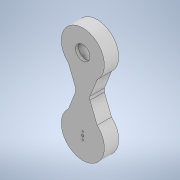
# Autodesk Inventor part: 2ndArm
Saved by Autodesk Inventor 2022 (Build 260153000, 153)
## iProperties
Created: 2022-02-11
Part Number: 2ndArm
Material: Generic
Document SubType Name: Modeling
Designer: Alexa
Density: 1 g/cm^3
Appearance: Default
Author: Alexa
Autodesk Inventor part; units mm, degrees
ref_plane "YZ Plane" through (0, 0, 0) normal (1, 0, 0) x (0, 1, 0)
ref_plane "XZ Plane" through (0, 0, 0) normal (0, 1, 0) x (-1, 0, 0)
ref_plane "XY Plane" through (0, 0, 0) normal (0, 0, 1) x (1, 0, 0)
sketch "Sketch1" plane through (0, 0, 0) normal (0, 0, 1) x (1, 0, 0)
  circle A0 centre (0, 0) radius 30
  circle A1 centre (0, 100) radius 30
  line L0 (-20, 0) -> (20, 0)
  line L1 (20, 0) -> (20, 100)
  line L2 (20, 100) -> (-20, 100)
  line L3 (-20, 100) -> (-20, 0)
  point P0 (20, 77.6393)
  point P1 (-20, 77.6393)
  point P2 (-20, 22.3607)
  point P3 (20, 22.3607)
  dimension "d0" = 60
  dimension "d1" = 60
  dimension "d2" = 40
  constraints: 8 end point, 2 centre point, 2 parallel, 1 coincident, 1 horizontal, 1 perpendicular
  measures "d0" diameter of A0
  measures "d1" diameter of A1
  measures "d2" distance of L2.end L1.end
extrude "Extrusion1" add sketch "Sketch1" along normal blind 20
sketch "Sketch2" plane through (0, 0, 20) normal (0, 0, 1) x (1, 0, 0)
  circle A0 centre (0, 0) radius 10
  dimension "d5" = 20
  constraints: 1 centre point, 1 coincident
  measures "d5" diameter of A0
extrude "Extrusion2" cut sketch "Sketch2" against normal blind 16
sketch "Sketch3" plane through (0, 0, 4) normal (0, 0, 1) x (1, 0, 0)
  circle A0 centre (0, 0) radius 1
  circle A1 centre (5, 0) radius 1
  circle A2 centre (-5, 0) radius 1
  dimension "d11" = 2
  dimension "d12" = 2
  dimension "d13" = 2
  constraints: 3 centre point, 1 coincident
  measures "d11" diameter of A0
  measures "d12" diameter of A1
  measures "d13" diameter of A2
extrude "Extrusion3" cut sketch "Sketch3" against normal blind 28.45
sketch "Sketch4" plane through (0, 0, 0) normal (0, 0, -1) x (-1, 0, 0)
  line L0 (0, 100) -> (10, 100)
  line L1 (10, 100) -> (10, 70)
  line L2 (10, 70) -> (0, 70)
  line L3 (0, 70) -> (0, 100)
  line L4 (0, 100) -> (-10, 100)
  line L5 (-10, 100) -> (-10, 70)
  line L6 (-10, 70) -> (0, 70)
  line L7 (0, 70) -> (0, 100)
  line L8 (10, 100) -> (-10, 100)
  line L9 (-10, 100) -> (-10, 110.5)
  line L10 (-10, 110.5) -> (10, 110.5)
  line L11 (10, 110.5) -> (10, 100)
  point P0 (0, 0)
  dimension "d16" = 10
  dimension "d17" = 30
  dimension "d18" = 10
  dimension "d19" = 10.5
  constraints: 24 end point, 6 parallel, 3 horizontal, 3 perpendicular, 2 point on line
  measures "d16" distance of L1.end L2.end
  measures "d17" distance of L0.end L1.end
  measures "d18" distance of L6.end L5.end
  measures "d19" distance of L8.end L9.end
extrude "Extrusion4" cut sketch "Sketch4" against normal blind 16
sketch "Sketch5" plane through (0, 0, 0) normal (0, 0, -1) x (-1, 0, 0)
  line L0 (10, 110.5) -> (10, 70) projected
  line L1 (10, 110.5) -> (-10, 110.5)
  line L2 (-10, 110.5) -> (-10, 118.1)
  line L3 (-10, 118.1) -> (10, 118.1)
  line L4 (10, 118.1) -> (10, 110.5)
  line L5 (10, 70) -> (-10, 70)
  line L6 (-10, 70) -> (-10, 62.4)
  line L7 (-10, 62.4) -> (10, 62.4)
  line L8 (10, 62.4) -> (10, 70)
  line L9 (-10, 110.5) -> (10, 110.5) projected
  line L10 (10, 110.5) -> (-10, 110.5)
  line L11 (-10, 110.5) -> (-10, 114.6)
  line L12 (-10, 114.6) -> (10, 114.6)
  line L13 (10, 114.6) -> (10, 110.5)
  line L14 (10, 70) -> (-10, 70)
  line L15 (-10, 70) -> (-10, 65.9)
  line L16 (-10, 65.9) -> (10, 65.9)
  line L17 (10, 65.9) -> (10, 70)
  line L18 (0, 110.5) -> (5, 110.5)
  line L19 (5, 110.5) -> (5, 114.6)
  line L20 (5, 114.6) -> (0, 114.6)
  line L21 (0, 114.6) -> (0, 110.5)
  line L22 (0, 110.5) -> (-5, 110.5)
  line L23 (-5, 110.5) -> (-5, 114.6)
  line L24 (-5, 114.6) -> (0, 114.6)
  line L25 (0, 114.6) -> (0, 110.5)
  line L26 (0, 70) -> (5, 70)
  line L27 (5, 70) -> (5, 65.9)
  line L28 (5, 65.9) -> (0, 65.9)
  line L29 (0, 65.9) -> (0, 70)
  line L30 (0, 70) -> (-5, 70)
  line L31 (-5, 70) -> (-5, 65.9)
  line L32 (-5, 65.9) -> (0, 65.9)
  line L33 (0, 65.9) -> (0, 70)
  point P0 (0, 0)
  dimension "d22" = 7.6
  dimension "d23" = 7.6
  dimension "d24" = 4.1
  dimension "d25" = 4.1
  dimension "d26" = 5
  dimension "d27" = 5
  dimension "d28" = 5
  dimension "d29" = 5
  constraints: 64 end point, 16 parallel, 8 horizontal, 8 perpendicular, 7 point on line, 2 midpoint
  measures "d22" distance of L1.end L2.end
  measures "d23" distance of L6.end L5.end
  measures "d24" distance of L10.end L11.end
  measures "d25" distance of L15.end L14.end
  measures "d26" distance of L20.end L19.end
  measures "d27" distance of L23.end L24.end
  measures "d28" distance of L27.end L28.end
  measures "d29" distance of L32.end L31.end
extrude "Extrusion5" cut sketch "Sketch5" against normal blind 10
sketch "Sketch6" plane through (0, 0, 10) normal (0, 0, -1) x (-1, 0, 0)
  line L0 (10, 110.5) -> (10, 70) projected
  line L1 (-10, 62.4) -> (-10, 118.1) projected
  line L2 (10, 110.5) -> (-10, 110.5)
  line L3 (-10, 110.5) -> (-10, 114.6)
  line L4 (-10, 114.6) -> (10, 114.6)
  line L5 (10, 114.6) -> (10, 110.5)
  line L6 (10, 70) -> (-10, 70) projected
  line L7 (-10, 62.4) -> (-10, 70) projected
  line L8 (10, 70) -> (-10, 70)
  line L9 (-10, 70) -> (-10, 65.9)
  line L10 (-10, 65.9) -> (10, 65.9)
  line L11 (10, 65.9) -> (10, 70)
  line L12 (-10, 110.5) -> (10, 110.5) projected
  line L13 (0, 114.6) -> (5, 114.6)
  line L14 (5, 114.6) -> (5, 110.5)
  line L15 (5, 110.5) -> (0, 110.5)
  line L16 (0, 110.5) -> (0, 114.6)
  line L17 (0, 110.5) -> (-5, 110.5)
  line L18 (-5, 110.5) -> (-5, 114.6)
  line L19 (-5, 114.6) -> (0, 114.6)
  line L20 (0, 114.6) -> (0, 110.5)
  line L21 (0, 70) -> (5, 70)
  line L22 (5, 70) -> (5, 65.9)
  line L23 (5, 65.9) -> (0, 65.9)
  line L24 (0, 65.9) -> (0, 70)
  line L25 (0, 70) -> (-5, 70)
  line L26 (-5, 70) -> (-5, 65.9)
  line L27 (-5, 65.9) -> (0, 65.9)
  line L28 (0, 65.9) -> (0, 70)
  circle A0 centre (5, 114.6) radius 1.35
  circle A1 centre (-5, 114.6) radius 1.35
  circle A2 centre (5, 65.9) radius 1.35
  circle A3 centre (-5, 65.9) radius 1.35
  point P0 (0, 0)
  dimension "d32" = 4.1
  dimension "d33" = 4.1
  dimension "d34" = 5
  dimension "d35" = 5
  dimension "d36" = 2.7
  dimension "d37" = 2.7
  dimension "d38" = 2.7
  dimension "d39" = 2.7
  constraints: 48 end point, 12 parallel, 8 point on line, 6 horizontal, 6 perpendicular, 4 centre point, 4 coincident, 2 midpoint
  measures "d32" distance of L2.end L3.end
  measures "d33" distance of L9.end L8.end
  measures "d34" distance of L14.end L15.end
  measures "d35" distance of L18.end L19.end
  measures "d36" diameter of A0
  measures "d37" diameter of A1
  measures "d38" diameter of A2
  measures "d39" diameter of A3
extrude "Extrusion6" cut sketch "Sketch6" against normal blind 8 contours A0 L4 L14 | L14 L4 A0 | L4 A0 | A2 L10 L22 | L22 L10 A2 | A2 L10 | A1 L4 L18 | L18 L4 A1 | L4 A1 | A3 L10 L26 | L26 L10 A3 | A3 L10
sketch "Sketch7" plane through (0, 0, 20) normal (0, 0, 1) x (1, 0, 0)
  circle A0 centre (0, 100) radius 10
  point P0 (0, 0)
  dimension "d50" = 20
  constraints: 1 centre point
  measures "d50" diameter of A0
extrude "Extrusion7" cut sketch "Sketch7" against normal blind 4
sketch "Sketch8" plane through (0, 0, 0) normal (0, 0, -1) x (-1, 0, 0)
  line L0 (20, 77.6393) -> (20, 22.3607) projected
  arc A0 (20, 77.6393) -> (-20, 77.6393) centre (0, 100) ccw projected
  line L1 (20, 22.3607) -> (-20, 22.3607)
  line L2 (-20, 22.3607) -> (-20, 77.6393)
  line L3 (-20, 77.6393) -> (20, 77.6393)
  line L4 (20, 77.6393) -> (20, 22.3607)
  line L5 (10, 118.1) -> (10, 62.4) projected
  line L6 (10, 77.6393) -> (-10, 77.6393)
  line L7 (-10, 77.6393) -> (-10, 47.6393)
  line L8 (-10, 47.6393) -> (10, 47.6393)
  line L9 (10, 47.6393) -> (10, 77.6393)
  line L10 (-10, 22.3607) -> (10, 22.3607)
  line L11 (10, 22.3607) -> (10, 52.3607)
  line L12 (10, 52.3607) -> (-10, 52.3607)
  line L13 (-10, 52.3607) -> (-10, 22.3607)
  line L14 (20, 77.6393) -> (10, 52.3607)
  line L15 (10, 47.6393) -> (20, 22.3607)
  line L16 (-20, 77.6393) -> (-10, 52.3607)
  line L17 (-10, 47.6393) -> (-20, 22.3607)
  point P0 (0, 0)
  dimension "d53" = 20
  dimension "d54" = 30
  dimension "d55" = 30
  constraints: 32 end point, 6 parallel, 5 point on line, 3 horizontal, 3 perpendicular
  measures "d53" distance of L8.end L7.end
  measures "d54" distance of L7.end L6.end
  measures "d55" distance of L11.end L10.end
extrude "Extrusion8" cut sketch "Sketch8" against normal blind 72.2 contours L0 L15 L9 L14 | L16 L7 L17 L2
sketch "Sketch9" plane through (0, 0, 20) normal (0, 0, 1) x (1, 0, 0)
  circle A0 centre (0, 0) radius 1 projected
  circle A1 centre (0, 0) radius 10
  constraints: 1 centre point, 1 coincident
extrude "Extrusion9" add sketch "Sketch9" against normal blind 20
sketch "Sketch10" plane through (0, 0, 0) normal (0, 0, -1) x (-1, 0, 0)
  circle A0 centre (0, 0) radius 1 projected
  circle A1 centre (0, 0) radius 10
  dimension "d60" = 20
  constraints: 1 centre point, 1 coincident
  measures "d60" diameter of A1
extrude "Extrusion10" cut sketch "Sketch10" against normal blind 16
sketch "Sketch11" plane through (0, 0, 16) normal (0, 0, -1) x (-1, 0, 0)
  circle A0 centre (0, 5) radius 1
  circle A1 centre (0, -5) radius 1
  point P0 (0, 0)
  dimension "d63" = 2
  dimension "d64" = 2
  constraints: 2 centre point
  measures "d63" diameter of A0
  measures "d64" diameter of A1
extrude "Extrusion11" cut sketch "Sketch11" against normal blind 22.1
chamfer "Chamfer2" distance 12 angle 45 1 edges at (10, 0, 0)
thread "Thread5" size "M3x0.5" class "6H" standard "ANSI Metric M Profile" full length
thread "Thread6" size "M3x0.5" class "6H" standard "ANSI Metric M Profile" full length
thread "Thread7" size "M3x0.5" class "6H" standard "ANSI Metric M Profile" full length
thread "Thread8" size "M3x0.5" class "6H" standard "ANSI Metric M Profile" full length
sketch "Sketch12" plane through (0, 0, 16) normal (0, 0, -1) x (-1, 0, 0)
  circle A0 centre (0, 0) radius 1 projected
  circle A1 centre (0, 0) radius 1.5
  dimension "d78" = 3
  constraints: 1 centre point, 1 coincident
  measures "d78" diameter of A1
extrude "Extrusion12" cut sketch "Sketch12" against normal blind 10
body "Solid1"
